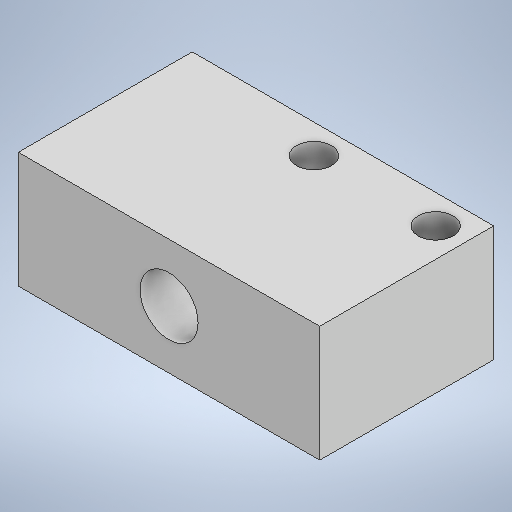
# Autodesk Inventor part: Steering
Saved by Autodesk Inventor 2025.2 (Build 292293000, 293)
## iProperties
Created: 2025-01-07
Part Number: Steering
Material: 일반
Document SubType Name: Modeling
Designer: SEON
Density: 1 g/cm^3
Appearance: 기본값
Author: SEON
Autodesk Inventor part; units mm, degrees
ref_plane "YZ Plane" through (0, 0, 0) normal (1, 0, 0) x (0, 1, 0)
ref_plane "XZ Plane" through (0, 0, 0) normal (0, 1, 0) x (-1, 0, 0)
ref_plane "XY Plane" through (0, 0, 0) normal (0, 0, 1) x (1, 0, 0)
sketch "스케치1" plane through (0, 0, 0) normal (0, 0, 1) x (1, 0, 0)
  line L0 (-13, -5) -> (13, -5)
  line L1 (13, -5) -> (13, 5)
  line L2 (13, 5) -> (-13, 5)
  line L3 (-13, 5) -> (-13, -5)
  line L4 (-13, -5) -> (13, 5) construction
  line L5 (13, -5) -> (-13, 5) construction
  point P0 (0, 0)
  dimension "d0" = 26
  dimension "d1" = 10
  constraints: 12 end point, 2 midpoint, 2 parallel, 1 horizontal, 1 perpendicular
  measures "d0" distance of L1.end L2.end
  measures "d1" distance of L2.end L0.start
extrude "돌출1" add sketch "스케치1" along normal blind 15
sketch "스케치2" plane through (-13, -5, 0) normal (0, -1, 0) x (1, 0, 0)
  circle A0 centre (13, 2.5) radius 1.5
  line L0 (0, 0) -> (26, 0) projected
  line L1 (0, 0) -> (0, 15) projected
  circle A1 centre (23.5, 2.5) radius 1.5
  line L2 (26, 0) -> (26, 15) projected
  point P0 (13, 0)
  point P1 (13, 0)
  point P2 (13, 0)
  dimension "d4" = 3
  dimension "d7" = 2.5
  dimension "d11" = 2.5
  dimension "d12" = 2.5
  constraints: 2 centre point, 2 midpoint, 1 equal radius, 1 vertical alignment
  measures "d4" diameter of A0
  measures "d7" distance of point (13, 0) A0.centre
  measures "d11" distance from line of L0 A1.centre
  measures "d12" distance from line of L2 A1.centre
extrude "돌출2" cut sketch "스케치2" against normal through all
sketch "스케치3" plane through (0, 0, 15) normal (0, 0, 1) x (1, 0, 0)
  circle A0 centre (0, 0) radius 2.5
  dimension "d8" = 5
  constraints: 1 centre point, 1 coincident
  measures "d8" diameter of A0
extrude "돌출3" cut sketch "스케치3" against normal blind 5
equation "\"d11\" = d7"
equation "\"d12\" = d11"
